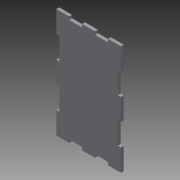
# Autodesk Inventor part: cajon abajo
Saved by Autodesk Inventor 2015 (Build 190159000, 159)
## iProperties
Created: 2016-01-26
Part Number: cajon abajo
Material: Generic
Document SubType Name: Modeling
Designer: iberopuebla
Density: 1 g/cm^3
Appearance: Default
Author: iberopuebla
Autodesk Inventor part; units mm, degrees
ref_plane "YZ Plane" through (0, 0, 0) normal (1, 0, 0) x (0, 1, 0)
ref_plane "XZ Plane" through (0, 0, 0) normal (0, 1, 0) x (-1, 0, 0)
ref_plane "XY Plane" through (0, 0, 0) normal (0, 0, 1) x (1, 0, 0)
sketch "Sketch1" plane through (0, 0, 0) normal (0, 1, 0) x (-1, 0, 0)
  line L0 (0, -132) -> (18, -132)
  line L1 (0, -264) -> (18, -264)
  line L2 (0, -396) -> (18, -396)
  line L3 (0, -528) -> (18, -528)
  line L4 (390, -132) -> (372, -132)
  line L5 (390, -264) -> (372, -264)
  line L6 (390, -396) -> (372, -396)
  line L7 (390, -528) -> (372, -528)
  line L8 (0, -132) -> (0, 0)
  line L9 (0, -660) -> (0, -528)
  line L10 (0, -396) -> (0, -264)
  line L11 (390, 0) -> (390, -132)
  line L12 (390, -264) -> (390, -396)
  line L13 (390, -528) -> (390, -660)
  line L14 (372, -132) -> (372, -264)
  line L15 (372, -396) -> (372, -528)
  line L16 (18, -396) -> (18, -528)
  line L17 (18, -132) -> (18, -264)
  line L18 (78, 0) -> (78, -18)
  line L19 (156, 0) -> (156, -18)
  line L20 (234, 0) -> (234, -18)
  line L21 (312, 0) -> (312, -18)
  line L22 (78, -642) -> (78, -660)
  line L23 (156, -642) -> (156, -660)
  line L24 (234, -642) -> (234, -660)
  line L25 (312, -642) -> (312, -660)
  line L26 (0, 0) -> (78, 0)
  line L27 (156, 0) -> (234, 0)
  line L28 (312, 0) -> (390, 0)
  line L29 (312, -18) -> (234, -18)
  line L30 (156, -18) -> (78, -18)
  line L31 (390, -660) -> (312, -660)
  line L32 (234, -660) -> (156, -660)
  line L33 (78, -660) -> (0, -660)
  line L34 (312, -642) -> (234, -642)
  line L35 (156, -642) -> (78, -642)
  dimension "d0" = 660
  dimension "d1" = 390
  dimension "d7" = 132
  dimension "d8" = 132
  dimension "d9" = 132
  dimension "d12" = 132
  dimension "d13" = 132
  dimension "d14" = 132
  dimension "d16" = 18
  dimension "d17" = 18
  dimension "d18" = 18
  dimension "d19" = 18
  dimension "d20" = 18
  dimension "d21" = 18
  dimension "d22" = 18
  dimension "d23" = 18
  dimension "d24" = 78
  dimension "d25" = 78
  dimension "d26" = 78
  dimension "d27" = 78
  dimension "d28" = 78
  dimension "d29" = 78
  dimension "d30" = 78
  dimension "d31" = 18
  dimension "d32" = 18
  dimension "d33" = 18
  dimension "d34" = 18
  dimension "d35" = 18
  dimension "d36" = 18
  dimension "d37" = 18
  dimension "d38" = 18
  dimension "d39" = 132
  dimension "d40" = 132
  constraints: 72 end point, 62 perpendicular, 19 parallel, 4 horizontal, 2 point on line
  measures "d0" distance of L11.start L13.end
  measures "d1" distance of L8.end L11.start
  measures "d7" distance between parallel lines of L0 L1
  measures "d8" distance between parallel lines of L2 L1
  measures "d9" distance between parallel lines of L3 L2
  measures "d12" distance between parallel lines of L5 L4
  measures "d13" distance between parallel lines of L6 L5
  measures "d14" distance between parallel lines of L7 L6
  measures "d16" horizontal distance of L11.start L4.end
  measures "d17" horizontal distance of L13.end L7.end
  measures "d18" distance of L6.start L6.end
  measures "d19" distance of L5.start L5.end
  measures "d20" distance of L1.start L1.end
  measures "d21" distance of L2.start L2.end
  measures "d22" horizontal distance of L9.start L3.end
  measures "d23" horizontal distance of L0.end L8.end
  measures "d24" distance between parallel lines of L8 L18
  measures "d25" distance between parallel lines of L18 L19
  measures "d26" distance between parallel lines of L19 L20
  measures "d27" distance between parallel lines of L21 L20
  measures "d28" distance between parallel lines of L23 L22
  measures "d29" distance between parallel lines of L24 L23
  measures "d30" distance between parallel lines of L25 L24
  measures "d31" vertical distance of L11.start L21.end
  measures "d32" vertical distance of L8.end L18.end
  measures "d33" distance of L20.start L20.end
  measures "d34" distance of L19.start L19.end
  measures "d35" distance of L23.start L23.end
  measures "d36" distance of L24.start L24.end
  measures "d37" vertical distance of L9.start L22.start
  measures "d38" vertical distance of L13.end L25.start
  measures "d39" vertical distance of L8.end L0.end
  measures "d40" distance between parallel lines of L28 L4
extrude "Extrusion1" add sketch "Sketch1" along normal blind 18
body "Solid1"
